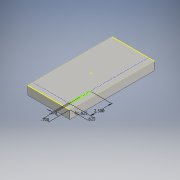
# Autodesk Inventor part: bottomOfCaseSmallTaps
Saved by Autodesk Inventor 2016 (Build 200138000, 138)
## iProperties
Created: 2015-09-19
Part Number: bottomOfCaseSmallTaps
Material: Generic
Document SubType Name: Modeling
Designer: steele
Density: 1 g/cm^3
Appearance: Default
Author: steele
Autodesk Inventor part; units mm, degrees
ref_plane "YZ Plane" through (0, 0, 0) normal (1, 0, 0) x (0, 1, 0)
ref_plane "XZ Plane" through (0, 0, 0) normal (0, 1, 0) x (-1, 0, 0)
ref_plane "XY Plane" through (0, 0, 0) normal (0, 0, 1) x (1, 0, 0)
sketch "Sketch1" plane through (0, 0, 0) normal (0, 1, 0) x (-1, 0, 0)
  line L0 (-63.5, 127) -> (-63.5, -127)
  line L1 (-63.5, -127) -> (63.5, -127)
  line L2 (63.5, -127) -> (63.5, 127)
  line L3 (63.5, 127) -> (-63.5, 127)
  line L4 (-63.5, 127) -> (63.5, -127) construction
  line L5 (-63.5, -127) -> (63.5, 127) construction
  point P0 (0, 0)
  dimension "height" = 127
  dimension "width" = 254
  constraints: 12 end point, 2 midpoint, 2 parallel, 1 perpendicular, 1 vertical
  measures "height" distance of L2.end L0.start
  measures "width" distance of L1.end L2.end
extrude "Extrusion1" add sketch "Sketch1" along normal blind 25.4
sketch "4-40" plane through (0, 25.4, 0) normal (0, 1, 0) x (1, 0, 0)
  line L0 (-63.5, -127) -> (63.5, -127) projected
  line L1 (45.72, -127) -> (45.72, 127) construction
  line L2 (63.5, 127) -> (-63.5, 127) projected
  line L3 (63.5, -127) -> (63.5, 127) construction
  line L4 (63.5, -111.125) -> (-63.5, -111.125) construction
  line L5 (-63.5, 127) -> (-63.5, -127) construction
  line L6 (48.26, -47.625) -> (48.26, -111.125)
  line L7 (48.26, -111.125) -> (43.18, -111.125)
  line L8 (43.18, -111.125) -> (43.18, -47.625)
  line L9 (43.18, -47.625) -> (48.26, -47.625)
  line L10 (48.26, -47.625) -> (43.18, -111.125) construction
  line L11 (48.26, -111.125) -> (43.18, -47.625) construction
  point P0 (0, 0)
  point P1 (45.72, -79.375)
  dimension "topFingerDistFromEdge" = 15.875
  dimension "d5" = 5.08
  dimension "d6" = 76.2
  dimension "d7" = 15.875
  dimension "d8" = 17.78
  constraints: 16 end point, 5 point on line, 2 midpoint, 2 parallel, 2 perpendicular, 1 vertical
  measures "topFingerDistFromEdge" distance between parallel lines of L0 L4
  measures "d5" distance between parallel lines of L8 L6
  measures "d7" distance from line of L7.end L0
  measures "d8" distance from line of point (45.72, -79.375) L3
equation "\"height\" = lowerCaseHeight"
equation "\"width\" = lowerCaseWidth"
equation "\"thickness\" = lowerCaseDepth"
equation "\"topFingerDistFromEdge\" = 0.5 * fingerWidth + fingerDistFromEdge"
equation "\"d6\" = tapLength4x40"
equation "\"fingerDistFromEdge\" = 6.35"
equation "\"fingerWidth\" = 19.05"
equation "\"tapDiam1d4x28\" = 5.08"
equation "\"tapDiam12x24\" = 5.08"
equation "\"tapDiam10x32\" = 5.08"
equation "\"tapDiam1d4x20\" = 5.08"
equation "\"tapDiam12x28\" = 5.08"
equation "\"tapDiam8x32\" = 5.08"
equation "\"tapDiam8x36\" = 5.08"
equation "\"tapDiam10x24\" = 5.08"
equation "\"tapDiam6x40\" = 5.08"
equation "\"lowerCaseHeight\" = 127"
equation "\"tapDiam6x32\" = 5.08"
equation "\"tapDiaam4x48\" = 5.08"
equation "\"lowerCaseDepth\" = 25.4"
equation "\"tapDiam4x40\" = 5.08"
equation "\"lowerCaseWidth\" = 254"
equation "\"tapLength6x32\" = 76.2"
equation "\"tapLength4x48\" = 76.2"
equation "\"tapLength4x40\" = 76.2"
body "Solid1"
